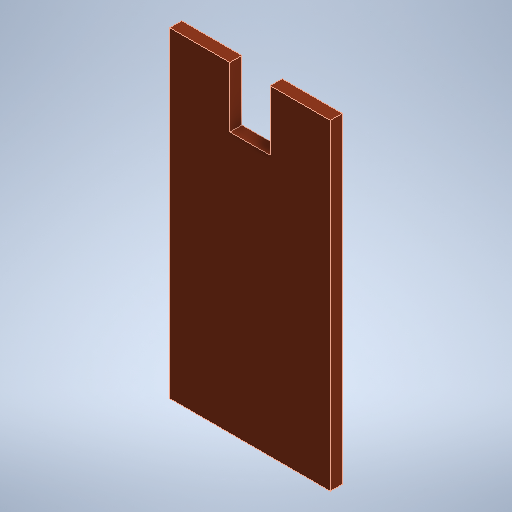
# Autodesk Inventor part: ramp extension
Saved by Autodesk Inventor 2025.4 (Build 294407000, 407)
## iProperties
Created: 2026-04-19
Part Number: ramp extension
Material: Generic
Document SubType Name: Sheet Metal
Designer: lenovo
Density: 1 g/cm^3
Sheet Metal Rule: Default_mm
Appearance: Default(1)
Author: lenovo
Autodesk Inventor part; units mm, degrees
ref_plane "YZ Plane" through (0, 0, 0) normal (1, 0, 0) x (0, 1, 0)
ref_plane "XZ Plane" through (0, 0, 0) normal (0, 1, 0) x (-1, 0, 0)
ref_plane "XY Plane" through (0, 0, 0) normal (0, 0, 1) x (1, 0, 0)
sketch "Sketch1" plane through (0, 0, 0) normal (0, 0, 1) x (1, 0, 0)
  line L0 (-20, -40) -> (20, -40)
  line L1 (20, -40) -> (20, 40)
  line L2 (20, 40) -> (-20, 40)
  line L3 (-20, 40) -> (-20, -40)
  line L4 (-20, -40) -> (20, 40) construction
  line L5 (20, -40) -> (-20, 40) construction
  line L6 (-5, 40) -> (5, 40)
  line L7 (5, 40) -> (5, 25)
  line L8 (5, 25) -> (-5, 25)
  line L9 (-5, 25) -> (-5, 40)
  line L10 (0, 40) -> (0, 0)
  dimension "d0" = 40
  dimension "d1" = 80
  dimension "d2" = 15
  dimension "d3" = 10
  measures "d0" distance of L2.end L1.end
  measures "d1" distance of L1.end L0.end
  measures "d2" distance of L6.end L7.end
  measures "d3" distance of L7.end L8.end
extrude "Plate1" add sketch "Sketch1" along normal blind 3 contours L3 L2 L9 L8 L7 L1 L0
equation "\"d4\" = Thickness"
equation "\"BendRadius\" = Thickness"
equation "\"BendReliefWidth\" = Thickness"
equation "\"BendReliefDepth\" = 0.5 * Thickness"
equation "\"CornerReliefSize\" = 4 * Thickness"
equation "\"MinimumRemnant\" = 2 * Thickness"
equation "\"TransitionRadius\" = BendRadius"
equation "\"JacobiRadiusSize\" = BendRadius"
equation "\"GapSize\" = Thickness"
equation "\"Thickness\" = 3"
body "Solid1"
